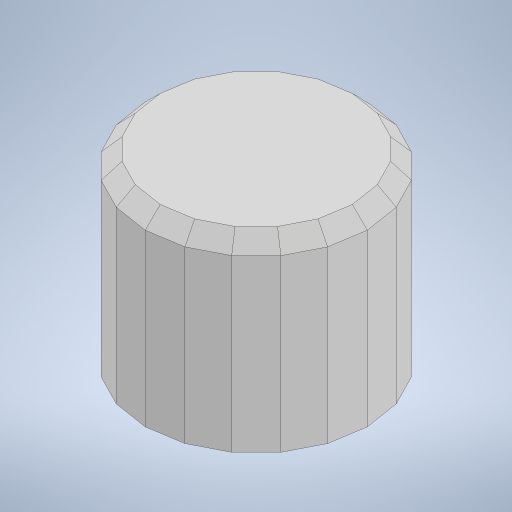
# Autodesk Inventor part: PotiBoxKnob
Saved by Autodesk Inventor 2024.3 (Build 283343000, 343)
## iProperties
Created: 2025-03-30
Part Number: PotiBoxKnob
Material: Generisch
Document SubType Name: Modeling
Designer: maxho
Density: 1 g/cm^3
Appearance: Vorgabe
Author: maxho
## iProperties of the stored document PotiBoxKnob_3D-Druck.ipt
Created: 2025-03-30
Part Number: PotiBoxKnob_3D-Druck
Material: Generisch
Document SubType Name: Modeling
Designer: maxho
Density: 1 g/cm^3
Appearance: Vorgabe
Author: maxho
Autodesk Inventor part; units mm, degrees
ref_plane "YZ Plane" through (0, 0, 0) normal (1, 0, 0) x (0, 1, 0)
ref_plane "XZ Plane" through (0, 0, 0) normal (0, 1, 0) x (-1, 0, 0)
ref_plane "XY Plane" through (0, 0, 0) normal (0, 0, 1) x (1, 0, 0)
sketch "Skizze1" plane through (0, 0, 0) normal (0, 0, 1) x (1, 0, 0)
  circle A0 centre (0, 0) radius 15 construction
  line L0 (-0.5, 19) -> (0.5, 19)
  line L1 (0.5, 19) -> (0.5, 14)
  line L2 (0.5, 14) -> (-0.5, 14)
  line L3 (-0.5, 14) -> (-0.5, 19)
  line L4 (0, -15) -> (-4.6353, -14.2658)
  line L5 (-4.6353, -14.2658) -> (-8.8168, -12.1353)
  line L6 (-8.8168, -12.1353) -> (-12.1353, -8.8168)
  line L7 (-12.1353, -8.8168) -> (-14.2658, -4.6353)
  line L8 (-14.2658, -4.6353) -> (-15, 0)
  line L9 (-15, 0) -> (-14.2658, 4.6353)
  line L10 (-14.2658, 4.6353) -> (-12.1353, 8.8168)
  line L11 (-12.1353, 8.8168) -> (-8.8168, 12.1353)
  line L12 (-8.8168, 12.1353) -> (-4.6353, 14.2658)
  line L13 (-4.6353, 14.2658) -> (0, 15)
  line L14 (0, 15) -> (4.6353, 14.2658)
  line L15 (4.6353, 14.2658) -> (8.8168, 12.1353)
  line L16 (8.8168, 12.1353) -> (12.1353, 8.8168)
  line L17 (12.1353, 8.8168) -> (14.2658, 4.6353)
  line L18 (14.2658, 4.6353) -> (15, 0)
  line L19 (15, 0) -> (14.2658, -4.6353)
  line L20 (14.2658, -4.6353) -> (12.1353, -8.8168)
  line L21 (12.1353, -8.8168) -> (8.8168, -12.1353)
  line L22 (8.8168, -12.1353) -> (4.6353, -14.2658)
  line L23 (4.6353, -14.2658) -> (0, -15)
  point P0 (0, 14)
  point P1 (-0.5, 14.9917)
  point P2 (0.5, 14.9917)
  point P3 (-0.5, 14.9208)
  point P4 (0.5, 14.9208)
  dimension "d0" = 30
  dimension "d3" = 1
  dimension "d4" = 1
  dimension "d12" = 5
  constraints: 48 end point, 2 coincident, 2 parallel, 2 vertical alignment, 1 horizontal, 1 midpoint, 1 perpendicular, 44 other
  measures "d3" length of L2
  measures "d4" distance of L0.start L0.end
  measures "d12" distance between parallel lines of L0 L2
extrude "Extrusion1" add sketch "Skizze1" along normal blind 25 contours L3 L2 L1 L14 L15 L16 L17 L18 L19 L20 L21 L22 L23 L4 L5 L6 L7 L8 L9 L10 L11 L12 L13
sketch "Skizze2" plane through (0, 0, 0) normal (0, 0, -1) x (-1, 0, 0)
  point P0 (0, 0)
  point P1 (0, 0)
  constraints: 1 coincident
hole "Bohrung1" at (0, 0, 0) direction (0, 0, 1) diameter 6.34 depth 20.62 counterbore diameter 10.525 counterbore depth 8.9375
sketch "Skizze3" plane through (0, 0, 20.62) normal (0, 0, -1) x (-1, 0, 0)
  line L0 (-3.17, 0.25) -> (3.17, 0.25)
  line L1 (3.17, 0.25) -> (3.17, -0.25)
  line L2 (3.17, -0.25) -> (-3.17, -0.25)
  line L3 (-3.17, -0.25) -> (-3.17, 0.25)
  line L4 (-3.17, 0.25) -> (3.17, -0.25) construction
  line L5 (3.17, 0.25) -> (-3.17, -0.25) construction
  circle A0 centre (0, 0) radius 3.17 projected
  circle A1 centre (0, 0) radius 3.17 projected
  point P0 (3.17, 0)
  dimension "d13" = 0.5
  constraints: 12 end point, 3 midpoint, 2 parallel, 1 horizontal, 1 horizontal alignment, 1 perpendicular, 1 other
  measures "d13" distance between parallel lines of L0 L2
extrude "Extrusion2" add sketch "Skizze3" along normal blind 0.5 contours L0 A0 L3 | L0 A0 L2 | A0 L2 L3 | L0 L1 A0 | L1 L2 A0
chamfer "Fasen1" distance 2 angle 45 20 edges at (13.2006, -6.726, 25) (14.6329, -2.3176, 25) (14.6329, 2.3176, 25) (13.2006, 6.726, 25) (10.476, 10.476, 25) (6.726, 13.2006, 25) (2.5676, 14.5933, 25) (-2.5676, 14.5933, 25) (-6.726, 13.2006, 25) (-10.476, 10.476, 25) (-13.2006, 6.726, 25) (-14.6329, 2.3176, 25) (-14.6329, -2.3176, 25) (-13.2006, -6.726, 25) (-10.476, -10.476, 25) (-6.726, -13.2006, 25) (-2.3176, -14.6329, 25) (2.3176, -14.6329, 25) (6.726, -13.2006, 25) (10.476, -10.476, 25)
equation "\"d0\" = KnobDiameter"
equation "\"d1\" = KnobHeight"
equation "\"d5\" = PotiShaftDiameter"
equation "\"KnobDiameter\" = 30"
equation "\"KnobHeight\" = 25"
equation "\"PotiShaftDiameter\" = 6.34"
